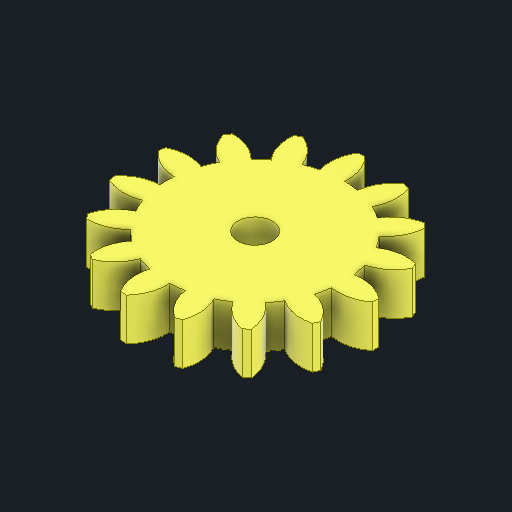
# Autodesk Inventor part: Gear
Saved by Autodesk Inventor 2024.1 (Build 281209000, 209)
## iProperties
Created: 2023-05-15
Part Number: Gear
Material: ABS Plastic
Document SubType Name: Modeling
Designer: jaege
Density: 1.06 g/cm^3
Appearance: Smooth - Yellow
Mass: 2.60043 g
Surface Area: 20.9715 cm^2
Volume: 2.45323 cm^3
Author: jaege
## iProperties of the stored document Gear_3DPrint.ipt
Created: 2023-05-15
Part Number: Gear_3DPrint
Material: Generic
Document SubType Name: Modeling
Designer: jaege
Density: 1 g/cm^3
Appearance: Default
Author: jaege
Autodesk Inventor part; units mm, degrees
ref_plane "YZ Plane" through (0, 0, 0) normal (1, 0, 0) x (0, 1, 0)
ref_plane "XZ Plane" through (0, 0, 0) normal (0, 1, 0) x (-1, 0, 0)
ref_plane "XY Plane" through (0, 0, 0) normal (0, 0, 1) x (1, 0, 0)
sketch "Sketch1" plane through (0, 0, 0) normal (0, 1, 0) x (-1, 0, 0)
  circle A0 centre (0, 0) radius 2.4765
  circle A1 centre (-8.1903, -11.4773) radius 6 construction
  circle A2 centre (0, -14.1) radius 6 construction
  line L0 (0, -14.1) -> (-8.1903, -11.4773) construction
  circle A3 centre (-8.1903, -11.4773) radius 5.3 construction
  circle A4 centre (0, -14.1) radius 5.3 construction
  line L1 (-4.7712, -16.4078) -> (-5.6471, -16.1273)
  circle A5 centre (0, 0) radius 12.5 construction
  line L2 (-8.1903, -11.4773) -> (0, 0) construction
  arc A6 (-4.7712, -16.4078) -> (-2.2465, -12.2965) centre (-8.1903, -11.4773) ccw
  arc A7 (-5.3141, -11.3142) -> (-5.6471, -16.1273) centre (0, -14.1) ccw
  line L3 (2.3149, -16.9299) -> (1.4006, -17.0299)
  arc A8 (2.3149, -16.9299) -> (2.9491, -12.1471) centre (-2.814, -13.8163) ccw
  arc A9 (-0.2527, -12.4974) -> (1.4006, -17.0299) centre (5.735, -12.881) ccw
  line L4 (9.0008, -14.5246) -> (8.2062, -14.9879)
  arc A10 (9.0008, -14.5246) -> (7.6348, -9.8974) centre (3.0489, -13.7664) ccw
  arc A11 (4.8523, -11.5198) -> (8.2062, -14.9879) centre (10.4783, -9.4347) ccw
  line L5 (14.1303, -9.6079) -> (13.5929, -10.3543)
  arc A12 (14.1303, -9.6079) -> (11.0004, -5.9364) centre (8.3846, -11.3361) ccw
  arc A13 (9.1183, -8.5502) -> (13.5929, -10.3543) centre (13.4099, -4.3571) ccw
  line L6 (16.8166, -3.03) -> (16.6292, -3.9304)
  arc A14 (16.8166, -3.03) -> (12.4639, -0.9489) centre (12.2706, -6.9458) ccw
  arc A15 (11.8077, -4.1023) -> (16.6292, -3.9304) centre (14.0228, 1.4739) ccw
  line L7 (16.5951, 4.0719) -> (16.7902, 3.1731)
  arc A16 (16.5951, 4.0719) -> (11.7723, 4.2027) centre (14.0348, -1.3544) ccw
  arc A17 (12.4554, 1.055) -> (16.7902, 3.1731) centre (12.211, 7.05) ccw
  line L8 (13.5042, 10.4697) -> (14.048, 9.7279)
  arc A18 (13.5042, 10.4697) -> (9.0451, 8.6276) centre (13.3723, 4.4712) ccw
  arc A19 (10.9495, 6.0298) -> (14.048, 9.7279) centre (8.2878, 11.4071) ccw
  line L9 (8.0783, 15.0572) -> (8.8768, 14.6007)
  arc A20 (8.0783, 15.0572) -> (4.754, 11.5607) centre (10.3976, 9.5236) ccw
  arc A21 (7.5503, 9.9621) -> (8.8768, 14.6007) centre (2.9316, 13.7919) ccw
  line L10 (1.2556, 17.0412) -> (2.1707, 16.949)
  arc A22 (1.2556, 17.0412) -> (-0.3592, 12.4948) centre (5.6251, 12.9294) ccw
  arc A23 (2.8456, 12.1718) -> (2.1707, 16.949) centre (-2.9316, 13.7919) ccw
  line L11 (-5.7843, 16.0786) -> (-4.9107, 16.3665)
  arc A24 (-5.7843, 16.0786) -> (-5.4102, 11.2685) centre (-0.1201, 14.0995) ccw
  arc A25 (-2.3511, 12.2769) -> (-4.9107, 16.3665) centre (-8.2878, 11.4071) ccw
  line L12 (-11.824, 12.3359) -> (-11.1431, 12.9542)
  arc A26 (-11.824, 12.3359) -> (-9.5258, 8.0938) centre (-5.8445, 12.8317) ccw
  arc A27 (-7.1413, 10.2592) -> (-11.1431, 12.9542) centre (-12.211, 7.05) ccw
  line L13 (-15.8192, 6.4601) -> (-15.4486, 7.302)
  arc A28 (-15.8192, 6.4601) -> (-11.9943, 3.5195) centre (-10.5583, 9.3452) ccw
  arc A29 (-10.6967, 6.4676) -> (-15.4486, 7.302) centre (-14.0228, 1.4739) ccw
  line L14 (-17.0791, -0.5326) -> (-17.083, 0.3871)
  arc A30 (-17.0791, -0.5326) -> (-12.3888, -1.6633) centre (-13.4465, 4.2428) ccw
  arc A31 (-12.4026, 1.5577) -> (-17.083, 0.3871) centre (-13.4099, -4.3571) ccw
  line L15 (-15.3859, -7.4333) -> (-15.7636, -6.5946)
  arc A32 (-15.3859, -7.4333) -> (-10.6413, -6.5585) centre (-14.0097, -1.5932) ccw
  arc A33 (-11.9639, -3.6216) -> (-15.7636, -6.5946) centre (-10.4783, -9.4347) ccw
  arc A34 (-2.2465, -12.2965) -> (-0.2527, -12.4974) centre (0, 0) ccw
  arc A35 (2.9491, -12.1471) -> (4.8523, -11.5198) centre (0, 0) ccw
  arc A36 (7.6348, -9.8974) -> (9.1183, -8.5502) centre (0, 0) ccw
  arc A37 (11.0004, -5.9364) -> (11.8077, -4.1023) centre (0, 0) ccw
  arc A38 (12.4639, -0.9489) -> (12.4554, 1.055) centre (0, 0) ccw
  arc A39 (11.7723, 4.2027) -> (10.9495, 6.0298) centre (0, 0) ccw
  arc A40 (9.0451, 8.6276) -> (7.5503, 9.9621) centre (0, 0) ccw
  arc A41 (4.754, 11.5607) -> (2.8456, 12.1718) centre (0, 0) ccw
  arc A42 (-0.3592, 12.4948) -> (-2.3511, 12.2769) centre (0, 0) ccw
  arc A43 (-5.4102, 11.2685) -> (-7.1413, 10.2592) centre (0, 0) ccw
  arc A44 (-9.5258, 8.0938) -> (-10.6967, 6.4676) centre (0, 0) ccw
  arc A45 (-11.9943, 3.5195) -> (-12.4026, 1.5577) centre (0, 0) ccw
  arc A46 (-12.3888, -1.6633) -> (-11.9639, -3.6216) centre (0, 0) ccw
  arc A47 (-10.6413, -6.5585) -> (-9.4565, -8.1746) centre (0, 0) ccw
  line L16 (-11.0323, -13.0486) -> (-11.7185, -12.4361)
  arc A48 (-11.0323, -13.0486) -> (-7.0537, -10.3196) centre (-12.1505, -7.1537) ccw
  arc A49 (-9.4565, -8.1746) -> (-11.7185, -12.4361) centre (-5.735, -12.881) ccw
  arc A50 (-7.0537, -10.3196) -> (-5.3141, -11.3142) centre (0, 0) ccw
  point P0 (4.8523, -11.5198)
  point P1 (9.1183, -8.5502)
  point P2 (11.8077, -4.1023)
  point P3 (12.4554, 1.055)
  point P4 (10.9495, 6.0298)
  point P5 (7.5503, 9.9621)
  point P6 (2.8456, 12.1718)
  point P7 (-2.3511, 12.2769)
  point P8 (-7.1413, 10.2592)
  point P9 (-10.6967, 6.4676)
  point P10 (-12.4026, 1.5577)
  point P11 (-11.9639, -3.6216)
  point P12 (-9.4565, -8.1746)
  point P13 (-2.2465, -12.2965)
  point P14 (-0.2527, -12.4974)
  point P15 (2.9491, -12.1471)
  point P16 (4.8523, -11.5198)
  point P17 (7.6348, -9.8974)
  point P18 (9.1183, -8.5502)
  point P19 (11.0004, -5.9364)
  point P20 (11.8077, -4.1023)
  point P21 (12.4639, -0.9489)
  point P22 (12.4554, 1.055)
  point P23 (11.7723, 4.2027)
  point P24 (10.9495, 6.0298)
  point P25 (9.0451, 8.6276)
  point P26 (7.5503, 9.9621)
  point P27 (4.754, 11.5607)
  point P28 (2.8456, 12.1718)
  point P29 (-0.3592, 12.4948)
  point P30 (-2.3511, 12.2769)
  point P31 (-5.4102, 11.2685)
  point P32 (-7.1413, 10.2592)
  point P33 (-9.5258, 8.0938)
  point P34 (-10.6967, 6.4676)
  point P35 (-11.9943, 3.5195)
  point P36 (-12.4026, 1.5577)
  point P37 (-12.3888, -1.6633)
  point P38 (-11.9639, -3.6216)
  point P39 (-10.6413, -6.5585)
  point P40 (-5.3141, -11.3142)
  point P41 (-9.4565, -8.1746)
  point P42 (-7.0537, -10.3196)
  dimension "d3" = 10.6
  dimension "d0" = 4.953
  dimension "d1" = 12
  dimension "d2" = 8.6
  dimension "d4" = 25
  dimension "d5" = 14.1
  dimension "d6" = 14.1
  dimension "d9" = 360
  dimension "d13" = 360
  constraints: 98 point on circle, 49 centre point, 34 end point, 19 coincident, 2 concentric, 2 equal radius, 1 vertical alignment, 233 other
  measures "d0" diameter of A0
  measures "d1" diameter of A2
  measures "d2" distance of L0.start L0.end
  measures "d4" diameter of A5
  measures "d5" distance of point (0, 0) L0.start
  measures "d6" distance of L2.start L2.end
extrude "Extrusion1" add sketch "Sketch1" along normal blind 6
body "Solid1"
